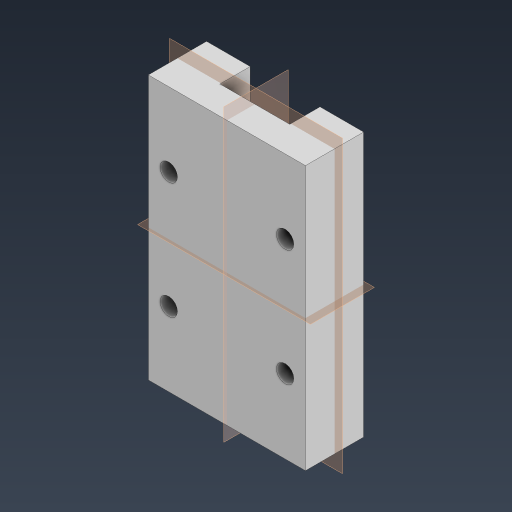
# Autodesk Inventor part: Каретка
Saved by Autodesk Inventor 2023.2 (Build 272271030, 271C)
## iProperties
Created: 2026-01-04
Part Number: Каретка
Material: Типовые
Document SubType Name: Modeling
Designer: Олег Коноваленко
Density: 1 g/cm^3
Appearance: По умолчанию
Author: Олег Коноваленко
Autodesk Inventor part; units mm, degrees
sketch "Эскиз1" plane through (0, 0, 0) normal (0, 1, 0) x (-1, 0, 0)
  line L0 (-13.5, -5) -> (13.5, -5)
  line L1 (13.5, -5) -> (13.5, 5)
  line L2 (13.5, 5) -> (-13.5, 5)
  line L3 (-13.5, 5) -> (-13.5, -5)
  line L4 (-13.5, -5) -> (13.5, 5) construction
  line L5 (13.5, -5) -> (-13.5, 5) construction
  line L6 (-6, -5) -> (6, -5)
  line L7 (6, -5) -> (6, 0.2)
  line L8 (6, 0.2) -> (-6, 0.2)
  line L9 (-6, 0.2) -> (-6, -5)
  line L10 (0, -7) -> (0, 7) construction
  point P0 (0, 0)
  point P1 (0, 0.2)
  dimension "d0" = 27
  dimension "d1" = 10
  dimension "d2" = 12
  dimension "d3" = 5.2
  constraints: 20 end point, 4 parallel, 3 midpoint, 2 horizontal, 2 perpendicular, 2 point on line
  measures "d0" distance of L1.end L2.end
  measures "d1" distance of L2.end L0.start
  measures "d2" distance of L7.end L8.end
  measures "d3" distance of L8.end L6.start
extrude "Выдавливание1" add sketch "Эскиз1" along normal mid plane 45.4 contours L3 L2 L1 L0 L7 L8 L9
sketch "Эскиз2" plane through (-13.5, 22.7, 5) normal (0, 0, 1) x (1, 0, 0)
  circle A0 centre (3.5, -12.7) radius 1.5
  circle A1 centre (3.5, -32.7) radius 1.5
  circle A2 centre (23.5, -12.7) radius 1.5
  circle A3 centre (23.5, -32.7) radius 1.5
  line L0 (3.5, -12.7) -> (3.5, -32.7) construction
  line L1 (3.5, -32.7) -> (23.5, -12.7) construction
  line L2 (23.5, -12.7) -> (3.5, -12.7) construction
  line L3 (23.5, -32.7) -> (23.5, -12.7) construction
  line L4 (3.5, -32.7) -> (23.5, -32.7) construction
  line L5 (23.5, -32.7) -> (3.5, -12.7) construction
  point P0 (13.5, -22.7)
  point P1 (13.5, -22.7)
  dimension "d6" = 3
  dimension "d7" = 20
  dimension "d8" = 20
  constraints: 12 end point, 4 centre point, 3 equal radius, 2 perpendicular, 1 coincident, 1 horizontal, 1 midpoint, 1 parallel
  measures "d6" diameter of A0
  measures "d7" distance of L0.start L0.end
  measures "d8" distance of L1.end L0.start
extrude "Выдавливание2" cut sketch "Эскиз2" against normal blind 5
